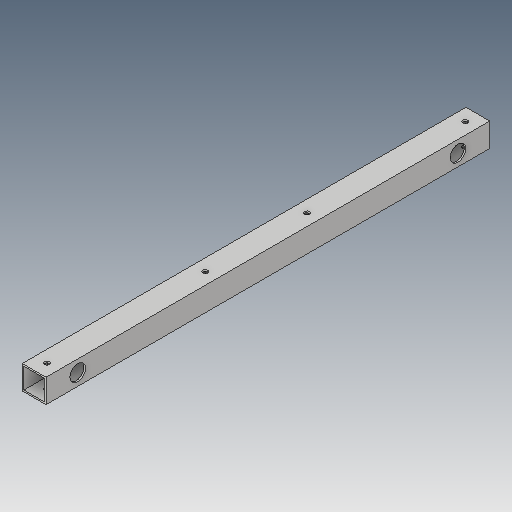
# Autodesk Inventor part: BaseSlideSTOPPERsq2
Saved by Autodesk Inventor 2019.4 (Build 234330000, 330)
## iProperties
Created: 2019-07-02
Part Number: BaseSlideSTOPPERsq2
Material: Generic
Document SubType Name: Modeling
Designer: AzLIer
Density: 1 g/cm^3
Appearance: Default
Author: AzLIer
Autodesk Inventor part; units mm, degrees
ref_plane "YZ Plane" through (0, 0, 0) normal (1, 0, 0) x (0, 1, 0)
ref_plane "XZ Plane" through (0, 0, 0) normal (0, 1, 0) x (-1, 0, 0)
ref_plane "XY Plane" through (0, 0, 0) normal (0, 0, 1) x (1, 0, 0)
sketch "スケッチ1" plane through (0, 0, 0) normal (0, 0, 1) x (1, 0, 0)
  line L0 (7.5, -7.5) -> (-7.5, -7.5)
  line L1 (-7.5, -7.5) -> (-7.5, 7.5)
  line L2 (-7.5, 7.5) -> (7.5, 7.5)
  line L3 (7.5, 7.5) -> (7.5, -7.5)
  line L4 (7.5, -7.5) -> (-7.5, 7.5) construction
  line L5 (-7.5, -7.5) -> (7.5, 7.5) construction
  point P0 (0, 0)
  dimension "d0" = 15
  dimension "d1" = 15
  constraints: 12 end point, 2 midpoint, 2 parallel, 1 horizontal, 1 perpendicular
  measures "d0" distance of L1.end L2.end
  measures "d1" distance of L0.end L1.end
extrude "押し出し1" add sketch "スケッチ1" along normal blind 280
shell "シェル1" thickness 1 removed faces 2 at (2.5, -2.5, 0) at (2.5, -2.5, 280)
sketch "スケッチ2" plane through (-7.5, 7.5, 0) normal (0, 1, 0) x (1, 0, 0)
  line L0 (7.5, -172.043) -> (7.5, -107.957) construction
  line L1 (15, -280) -> (0, -280) projected
  line L2 (0, 0) -> (0, -280) projected
  line L3 (0, -140) -> (7.5, -140) construction
  point P0 (7.5, 0)
  point P1 (7.5, -280)
  point P2 (7.5, -272)
  point P3 (7.5, -8)
  dimension "d5" = 64.086
  dimension "d29" = 264
  constraints: 4 end point, 3 midpoint, 2 coincident, 2 point on line, 1 horizontal alignment, 1 perpendicular, 1 symmetric about line, 1 vertical, 1 vertical alignment
  measures "d5" distance of L0.start L0.end
  measures "d29" distance of point (7.5, -8) point (7.5, -272)
hole "穴1" at (0, 7.5, 172.043) at (0, 7.5, 107.957) at (0, 7.5, 272) at (0, 7.5, 8) direction (0, -1, 0) diameter 3.2 end through all
sketch "スケッチ3" plane through (-7.5, -7.5, 0) normal (-1, 0, 0) x (0, 0, 1)
  line L0 (20, 7.5) -> (260, 7.5)
  line L1 (0, 15) -> (280, 15) projected
  line L2 (280, 15) -> (280, 0) projected
  point P0 (0, 7.5)
  point P1 (140, 7.5)
  point P2 (140, 15)
  point P3 (280, 7.5)
  dimension "d13" = 240
  constraints: 3 midpoint, 2 end point, 1 horizontal, 1 horizontal alignment, 1 vertical alignment
  measures "d13" distance of L0.start L0.end
hole "穴2" at (-7.5, 0, 260) at (-7.5, 0, 20) direction (1, 0, 0) diameter 10 end through all
